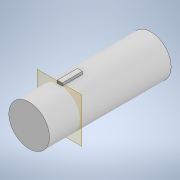
# Autodesk Inventor part: clutch03Shaft
Saved by Autodesk Inventor 2021 (Build 250183000, 183)
## iProperties
Created: 2020-07-05
Part Number: clutch03Shaft
Material: Generic
Document SubType Name: Modeling
Designer: robst
Density: 1 g/cm^3
Appearance: Default
Author: robst
Autodesk Inventor part; units mm, degrees
ref_plane "YZ Plane" through (0, 0, 0) normal (1, 0, 0) x (0, 1, 0)
ref_plane "XZ Plane" through (0, 0, 0) normal (0, 1, 0) x (-1, 0, 0)
ref_plane "XY Plane" through (0, 0, 0) normal (0, 0, 1) x (1, 0, 0)
sketch "Sketch1" plane through (0, 0, 0) normal (0, 0, 1) x (1, 0, 0)
  circle A0 centre (0, 0) radius 12.7
  dimension "d0" = 25.4
  constraints: 1 centre point, 1 coincident
  measures "d0" diameter of A0
extrude "Extrusion1" add sketch "Sketch1" against normal blind 76.2
ref_plane "Work Plane1" through (0, 0, -19.05) normal (0, 0, 1) x (1, 0, 0)
sketch "Sketch3" plane through (0, 0, -19.05) normal (0, 0, 1) x (1, 0, 0)
  circle A0 centre (0, 0) radius 12.7 projected
  arc A1 (1.5875, 14.199) -> (-1.5875, 14.199) centre (0, 0) ccw
  arc A2 (1.5875, 12.6004) -> (-1.5875, 12.6004) centre (0, 0) ccw
  line L0 (-1.5875, 12.6004) -> (-1.5875, 14.199)
  line L1 (1.5875, 12.6004) -> (1.5875, 14.199)
  line L2 (0, 0) -> (0, 14.2875) construction
  point P0 (-1.5875, 12.6004)
  point P1 (1.5875, 12.6004)
  dimension "d4" = 28.575
  dimension "d6" = 1.5875
  dimension "d7" = 1.5875
  constraints: 6 end point, 5 point on circle, 2 centre point, 2 coincident, 2 vertical, 1 concentric
  measures "d4" diameter of A1
  measures "d6" distance between parallel lines of L0 L2
  measures "d7" distance between parallel lines of L1 L2
extrude "Extrusion2" add sketch "Sketch3" against normal blind 12.7 contours A0 L0 A1 L1
body "Solid1"
